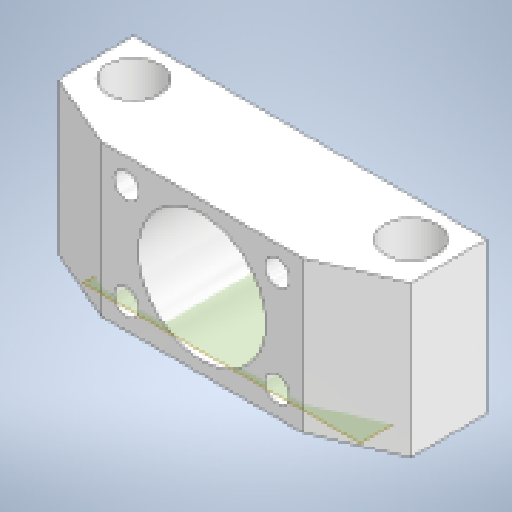
# Autodesk Inventor part: Motor Sleeve
Saved by Autodesk Inventor 2023.2 (Build 272271000, 271)
## iProperties
Created: 2023-04-12
Part Number: Motor Sleeve
Material: UHMW, White
Document SubType Name: Modeling
Designer: Nathan Cai
Density: 0.94 g/cm^3
Appearance: Smooth - White
Mass: 5.55755 g
Surface Area: 47.1476 cm^2
Volume: 5.91229 cm^3
Author: Nathan Cai
Autodesk Inventor part; units mm, degrees
ref_plane "YZ Plane" through (0, 0, 0) normal (1, 0, 0) x (0, 1, 0)
ref_plane "XZ Plane" through (0, 0, 0) normal (0, 1, 0) x (-1, 0, 0)
ref_plane "XY Plane" through (0, 0, 0) normal (0, 0, 1) x (1, 0, 0)
sketch "Sketch1" plane through (0, 0, 0) normal (0, 0, 1) x (1, 0, 0)
  line L0 (-12.7, -6.35) -> (12.7, -6.35) construction
  line L1 (12.7, -6.35) -> (12.7, 6.35) construction
  line L2 (12.7, 6.35) -> (-12.7, 6.35) construction
  line L3 (-12.7, 6.35) -> (-12.7, -6.35) construction
  line L4 (-12.7, -6.35) -> (12.7, 6.35) construction
  line L5 (12.7, -6.35) -> (-12.7, 6.35) construction
  circle A0 centre (0, 0) radius 11
  circle A1 centre (-12.7, 6.35) radius 1.5875
  circle A2 centre (12.7, 6.35) radius 1.5875
  circle A3 centre (-12.7, -6.35) radius 1.5875
  circle A4 centre (12.7, -6.35) radius 1.5875
  line L6 (-15.875, -9.525) -> (15.875, -9.525)
  line L7 (15.875, -9.525) -> (15.875, 9.525)
  line L8 (15.875, 9.525) -> (-15.875, 9.525)
  line L9 (-15.875, 9.525) -> (-15.875, -9.525)
  line L10 (-15.875, -9.525) -> (15.875, 9.525) construction
  line L11 (15.875, -9.525) -> (-15.875, 9.525) construction
  line L12 (9.525, -12.7) -> (-9.525, -12.7)
  line L13 (-9.525, -12.7) -> (-9.525, 12.7)
  line L14 (-9.525, 12.7) -> (9.525, 12.7)
  line L15 (9.525, 12.7) -> (9.525, -12.7)
  line L16 (9.525, -12.7) -> (-9.525, 12.7) construction
  line L17 (-9.525, -12.7) -> (9.525, 12.7) construction
  point P0 (-9.525, 9.525)
  point P1 (-5.5022, 9.525)
  point P2 (5.5022, 9.525)
  point P3 (9.525, 9.525)
  point P4 (9.525, -9.525)
  point P5 (5.5022, -9.525)
  point P6 (-5.5022, -9.525)
  point P7 (-9.525, -9.525)
  dimension "d0" = 25.4
  dimension "d1" = 12.7
  dimension "d2" = 22
  dimension "d3" = 3.175
  dimension "d6" = 25.4
  dimension "d9" = 12.7
  dimension "d12" = 31.75
  dimension "d13" = 19.05
  dimension "d42" = 19.05
  dimension "d43" = 25.4
  constraints: 36 end point, 6 midpoint, 6 parallel, 5 centre point, 4 horizontal, 3 perpendicular, 2 coincident, 1 vertical, 6 other
  measures "d0" distance of L2.end L1.end
  measures "d1" distance of L1.end L0.end
  measures "d2" diameter of A0
  measures "d3" diameter of A1
  measures "d6" distance of A1.centre A2.centre
  measures "d9" distance of A1.centre A3.centre
  measures "d12" distance of L8.end L7.end
  measures "d13" distance of L7.end L6.end
  measures "d42" distance of L13.end L14.end
  measures "d43" distance between parallel lines of L14 L12
extrude "Extrusion1" add sketch "Sketch1" along normal blind 13.625 contours A0 L15 L8 L7 L6 | A0 L8 L15 | L15 L6 A0 | A0 L8 L13 L14 L15 | L6 L15 L12 L13 A0 | A0 L13 L8 | L6 L13 A0 | A0 L13 L6 L9 L8
ref_plane "Work Plane1" through (-15.875, -6.35, 0) normal (0, -1, 0) x (1, 0, 0)
sketch "Sketch2" plane through (-15.875, -9.525, 0) normal (0, -1, 0) x (1, 0, 0)
  line L0 (0, 0) -> (0, 13.625) projected
  line L1 (0, 0) -> (-9.525, 0)
  line L2 (-9.525, 0) -> (-9.525, 9.525)
  line L3 (-9.525, 9.525) -> (0, 9.525)
  line L4 (0, 9.525) -> (0, 0)
  line L5 (-9.525, 9.525) -> (0, 0) construction
  circle A0 centre (-4.7625, 4.7625) radius 3.302
  line L6 (15.875, 0) -> (15.875, -6.35) construction
  line L7 (31.75, 0) -> (41.275, 0)
  line L8 (41.275, 0) -> (41.275, 9.525)
  line L9 (41.275, 9.525) -> (31.75, 9.525)
  line L10 (31.75, 9.525) -> (31.75, 0)
  line L11 (41.275, 9.525) -> (31.75, 0) construction
  circle A1 centre (36.5125, 4.7625) radius 3.302
  point P0 (0, 9.525)
  dimension "d38" = 9.525
  dimension "d39" = 9.525
  dimension "d40" = 6.604
  dimension "d41" = 6.35
  constraints: 22 end point, 5 symmetric about line, 2 centre point, 2 parallel, 1 horizontal, 1 midpoint, 1 perpendicular, 1 vertical, 1 other
  measures "d38" distance of L2.end L3.end
  measures "d39" distance of L1.end L2.end
  measures "d40" diameter of A0
  measures "d41" distance of L6.start L6.end
extrude "Extrusion2" add sketch "Sketch2" against normal blind 19.05
chamfer "Chamfer2" distance 4.1 distance2 9.525 1 edges at (-15.875, 0, 9.525) measured on face at (-15.875, 3.175, 12.2583)
chamfer "Chamfer3" distance 4.1 distance2 9.525 1 edges at (15.875, 0, 9.525) measured on face at (15.875, -3.175, 12.2583)
fillet "Fillet3" radius 1.5875 4 edges at (9.525, -12.7, 6.8125) (-9.525, -12.7, 6.8125) (-9.525, 12.7, 6.8125) (9.525, 12.7, 6.8125)
equation "\"d6\" = d0"
equation "\"d9\" = d1"
body "Solid1"
